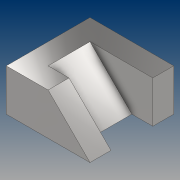
# Autodesk Inventor part: 48
Saved by Autodesk Inventor 2020.2 (Build 242310000, 310)
## iProperties
Created: 2020-09-17
Part Number: 48
Material: 鋼、碳鋼
Document SubType Name: Modeling
Designer: user
Density: 7.85 g/cm^3
Appearance: 半拋光
Mass: 172.7 g
Surface Area: 60.4853 cm^2
Volume: 22 cm^3
Author: user
Autodesk Inventor part; units mm, degrees
ref_plane "YZ Plane" through (0, 0, 0) normal (1, 0, 0) x (0, 1, 0)
ref_plane "XZ Plane" through (0, 0, 0) normal (0, 1, 0) x (-1, 0, 0)
ref_plane "XY Plane" through (0, 0, 0) normal (0, 0, 1) x (1, 0, 0)
sketch "草圖1" plane through (0, 0, 0) normal (0, 1, 0) x (-1, 0, 0)
  line L0 (0, -20) -> (-40, -20)
  line L1 (-40, -20) -> (-40, 20)
  line L2 (-40, 20) -> (0, 20)
  line L3 (0, 20) -> (0, -20)
  point P0 (0, 0)
  point P1 (0, 0)
  dimension "d0" = 40
  dimension "d1" = 40
  constraints: 8 end point, 2 parallel, 1 coincident, 1 horizontal, 1 midpoint, 1 perpendicular
  measures "d0" distance of L1.end L2.end
  measures "d1" distance of L2.end L0.start
extrude "擠出1" add sketch "草圖1" along normal blind 20
sketch "草圖2" plane through (0, 20, 0) normal (0, 1, 0) x (1, 0, 0)
  line L0 (0, 20) -> (40, 20) projected
  line L1 (40, 20) -> (40, -20) projected
  line L2 (40, -20) -> (0, -20) projected
  line L3 (0, -20) -> (0, 20) projected
  line L4 (10, 10) -> (40, 10)
  line L5 (40, 10) -> (40, -10)
  line L6 (40, -10) -> (10, -10)
  line L7 (10, -10) -> (10, 10)
  point P0 (0, 0)
  point P1 (40, 0)
  dimension "d4" = 20
  dimension "d5" = 30
  constraints: 8 end point, 2 midpoint, 2 parallel, 1 horizontal, 1 perpendicular
  measures "d4" distance of L6.end L4.start
  measures "d5" distance of L4.start L4.end
extrude "擠出2" cut sketch "草圖2" against normal through all contours L1 L6 L7 L4
sketch "草圖3" plane through (0, 0, 20) normal (0, 0, 1) x (1, 0, 0)
  line L0 (40, 0) -> (0, 0) projected
  line L1 (0, 0) -> (0, 20) projected
  line L2 (0, 20) -> (40, 20) projected
  line L3 (40, 20) -> (40, 0) projected
  line L4 (40, 0) -> (40, 20) projected
  line L5 (40, 0) -> (20, 20)
  dimension "d8" = 20
  constraints: 2 end point, 1 midpoint
  measures "d8" distance of L2.end L5.end
extrude "擠出3" cut sketch "草圖3" against normal blind 13 contours L5 L2 L3
sketch "草圖4" plane through (10, 20, -10) normal (0, 0, 1) x (1, 0, 0)
  line L0 (-10, 0) -> (0, 0) projected
  line L1 (0, 0) -> (30, 0) projected
  line L2 (30, 0) -> (30, -20) projected
  line L3 (30, -20) -> (0, -20) projected
  line L4 (0, -20) -> (-10, -20) projected
  line L5 (-10, -20) -> (-10, 0) projected
  line L6 (0, 0) -> (0, -20) projected
  line L7 (0, 0) -> (20, -20)
  line L8 (30, -20) -> (-10, -20) projected
  dimension "d11" = 30
  constraints: 2 end point, 1 point on line
  measures "d11" distance from line of L7.end L5
extrude "擠出4" add sketch "草圖4" along normal up to surface (20 mm away) contours L7 L3 L6
